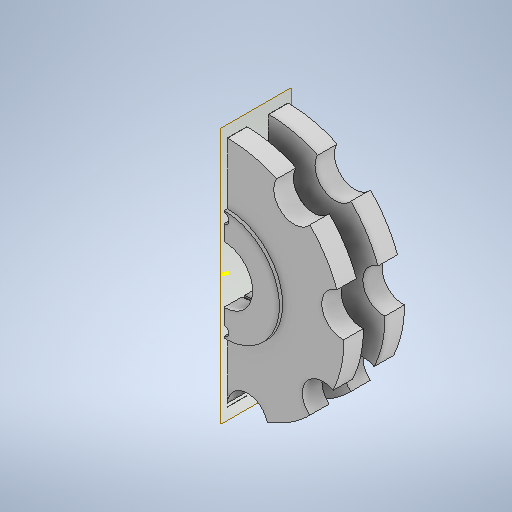
# Autodesk Inventor part: 59-01-002-C
Saved by Autodesk Inventor 2025.2 (Build 292293000, 293)
## iProperties
Created: 2024-11-14
Part Number: 59-01-002-C
Material: Generic
Document SubType Name: Modeling
Designer: Zvonko.Gabric
Density: 1 g/cm^3
Appearance: Default
Description: Stator
Author: Zvonko.Gabric
Autodesk Inventor part; units mm, degrees
ref_plane "XZ Plane" through (0, 0, 0) normal (0, 1, 0) x (-1, 0, 0)
ref_plane "XY Plane" through (0, 0, 0) normal (0, 0, 1) x (1, 0, 0)
sketch "Sketch1" plane through (0, 0, 0) normal (0, 1, 0) x (-1, 0, 0)
  line L0 (0, 0) -> (0, -37.3)
  line L1 (0, -37.3) -> (-71.75, -37.3)
  line L2 (-71.75, -37.3) -> (-71.75, -25.3)
  line L3 (-71.75, -25.3) -> (-41.05, -25.3)
  line L4 (-41.05, -25.3) -> (-41.05, -12)
  line L5 (-41.05, -12) -> (-71.75, -12)
  line L6 (-71.75, -12) -> (-71.75, 0)
  line L7 (-71.75, 0) -> (0, 0)
  dimension "d0" = 37.3
  dimension "d1" = 71.75
  dimension "d2" = 12
  dimension "d3" = 30.7
  dimension "d4" = 13.3
  constraints: 16 end point, 5 perpendicular, 2 point on line, 1 parallel, 1 vertical
  measures "d0" distance of L0.start L0.end
  measures "d1" distance of L0.end L1.end
  measures "d2" distance of L1.end L2.end
  measures "d3" distance of L2.end L3.end
  measures "d4" distance of L3.end L4.end
revolve "Revolution1" add sketch "Sketch1" angle 360 about axis through (0, 0, 0) along (0, 0, -1)
sketch "Sketch2" plane through (0, 0, 0) normal (0, 0, 1) x (1, 0, 0)
  circle A0 centre (0, 0) radius 34
  dimension "d6" = 68
  constraints: 1 centre point, 1 coincident
  measures "d6" diameter of A0
extrude "Extrusion1" add sketch "Sketch2" along normal blind 2
sketch "Sketch3" plane through (0, 0, 2) normal (0, 0, 1) x (1, 0, 0)
  circle A0 centre (0, 0) radius 17.5
  dimension "d9" = 35
  constraints: 1 centre point, 1 coincident
  measures "d9" diameter of A0
extrude "Extrusion2" cut sketch "Sketch3" against normal through all
sketch "Sketch4" plane through (0, 0, 2) normal (0, 0, 1) x (1, 0, 0)
  point P0 (0, 0)
sketch "Sketch7" plane through (0, 0, 0) normal (0, 0, 1) x (1, 0, 0)
  circle A0 centre (0, 0) radius 71.75
  circle A1 centre (-12.4593, 70.66) radius 12.5
  line L0 (-12.4593, 70.66) -> (0, 0) construction
  line L1 (0, 71.75) -> (0, 0) construction
  line L2 (-50.7349, 50.7349) -> (0, 0) construction
  circle A2 centre (-58.7742, 41.1541) radius 12.5
  line L3 (-71.75, 0) -> (0, 0) construction
  circle A3 centre (-70.66, -12.4593) radius 12.5
  line L4 (-50.7349, -50.7349) -> (0, 0) construction
  circle A4 centre (-41.1541, -58.7742) radius 12.5
  line L5 (0, -71.75) -> (0, 0) construction
  circle A5 centre (12.4593, -70.66) radius 12.5
  line L6 (50.7349, -50.7349) -> (0, 0) construction
  circle A6 centre (58.7742, -41.1541) radius 12.5
  line L7 (71.75, 0) -> (0, 0) construction
  circle A7 centre (70.66, 12.4593) radius 12.5
  line L8 (50.7349, 50.7349) -> (0, 0) construction
  circle A8 centre (41.1541, 58.7742) radius 12.5
  line L9 (41.1541, 58.7742) -> (0, 0) construction
  line L10 (70.66, 12.4593) -> (0, 0) construction
  dimension "d26" = 25
  dimension "d27" = 143.5
  dimension "d28" = 10
  dimension "d31" = 360
  constraints: 22 end point, 9 centre point, 3 coincident, 2 point on circle, 1 vertical, 39 other
  measures "d26" diameter of A1
  measures "d27" diameter of A0
  measures "d28" angle of L1 L0
extrude "Extrusion4" cut sketch "Sketch7" against normal through all contours A7 A0 | A0 A7 | A6 A0 | A0 A6 | A8 A0 | A0 A8 | A5 A0 | A0 A5 | A1 A0 | A0 A1 | A4 A0 | A0 A4 | A2 A0 | A0 A2 | A3 A0 | A0 A3
sketch "Sketch8" plane through (0, 0, 2) normal (0, 0, 1) x (1, 0, 0)
  arc A0 (30.3291, 65.0247) -> (-0.0069, 71.75) centre (0, 0) ccw projected
  line L0 (-0.0069, 71.75) -> (-0.0069, -34) construction
  circle A1 centre (0, 0) radius 34 projected
  circle A2 centre (-0.0069, 30) radius 3
  circle A3 centre (-0.0069, -30) radius 3
  dimension "d35" = 30
  dimension "d36" = 6
  dimension "d37" = 30
  dimension "d38" = 6
  constraints: 2 centre point, 2 end point, 2 point on line, 1 vertical, 2 other
  measures "d35" distance of point (0, 0) A3.centre
  measures "d36" diameter of A3
  measures "d37" distance of point (0, 0) A2.centre
  measures "d38" diameter of A2
extrude "Extrusion5" cut sketch "Sketch8" against normal blind 17 contours A2 | A3
thread "Thread1" size "M6x1" class "6H" standard "ANSI Metric M Profile" length 12
thread "Thread2" size "M6x1" class "6H" standard "ISO Metric profile" length 12 offset 5
thread "Thread3" size "M6x1" class "6H" standard "ISO Metric profile" length 12 offset 5
sketch "Sketch10" plane through (41.1541, 58.7742, 0) normal (0, 0, 1) x (0.819152, -0.5735764, 0)
  circle A0 centre (0, -71.75) radius 41.05 projected
  circle A1 centre (-17.2129, -47.1794) radius 3 projected
  line L0 (0, -71.75) -> (-17.2129, -47.1794) construction
  arc A2 (-41.1597, -130.5202) -> (-58.7702, -112.9097) centre (-50.7349, -122.4849) ccw projected
  line L1 (0, -71.75) -> (-50.7349, -122.4849) construction
  arc A3 (-37.3679, -113.3606) -> (-41.6106, -109.1179) centre (-39.4892, -111.2392) ccw
  arc A4 (-40.0331, -116.0257) -> (-44.2757, -111.7831) centre (-50.7349, -122.4849) ccw
  line L2 (-39.4892, -111.2392) -> (-37.3679, -113.3606) construction
  line L3 (-39.4892, -111.2392) -> (-41.6106, -109.1179) construction
  line L4 (-37.3679, -113.3606) -> (-40.0331, -116.0257)
  line L5 (-41.6106, -109.1179) -> (-44.2757, -111.7831)
  point P0 (-42.9431, -110.4505)
  point P1 (-44.2757, -111.7831)
  point P2 (-40.0331, -116.0257)
  dimension "d56" = 6
  dimension "d57" = 55
  dimension "d58" = 6
  constraints: 12 end point, 4 point on circle, 2 centre point, 1 coincident, 1 midpoint, 1 point on line, 1 tangent
  measures "d56" diameter of A3
  measures "d57" distance from line of L0 L2.start
  measures "d58" distance from line of point (-42.943, -110.451) L4
extrude "Extrusion7" cut sketch "Sketch10" against normal blind 13 contours A2 L5 A3 L4
sketch "Sketch11" plane through (-41.1541, -58.7742, 0) normal (0, 0, 1) x (0.819152, -0.5735764, 0)
  circle A0 centre (-17.2129, 96.3206) radius 3 projected
  line L0 (0, 71.75) -> (-17.2129, 96.3206) construction
  line L1 (0, 71.75) -> (-36.8559, 45.9306) construction
  circle A1 centre (-36.8559, 45.9306) radius 2.05
  dimension "d61" = 4.1
  dimension "d62" = 45
  constraints: 4 end point, 1 centre point, 1 coincident
  measures "d61" diameter of A1
  measures "d62" distance from line of L0 A1.centre
extrude "Extrusion8" cut sketch "Sketch11" against normal blind 8 contours A1
sketch "Sketch12" plane through (41.1541, 58.7742, -37.3) normal (0, 0, -1) x (-0.819152, 0.5735764, 0)
  circle A0 centre (0, -71.75) radius 31
  dimension "d65" = 62
  constraints: 1 centre point, 1 coincident
  measures "d65" diameter of A0
extrude "Extrusion9" cut sketch "Sketch12" against normal blind 5.5
chamfer "Chamfer1" distance 10 distance2 5.5 1 edges at (25.3937, -17.7809, -37.3) measured on face at (49.9559, -10.1171, -37.3)
sketch "Sketch13" plane through (-0.0069, 30, -15) normal (0, 0, 1) x (1, 0, 0)
  point P0 (0.0069, -30)
sketch "Sketch14" plane through (-0.0069, 30, -15) normal (0, 0, 1) x (1, 0, 0)
  point P0 (0.0069, -30)
ref_plane "Work Plane1" through (0, 0, 0) normal (1, 0, 0) x (0, 1, 0)
sketch "Sketch15" plane through (0, 0, 0) normal (1, 0, 0) x (0, 1, 0)
  point P0 (0, 0)
sketch "Sketch16" plane through (0, 0, 0) normal (1, 0, 0) x (0, 1, 0)
  line L0 (27, -15) -> (33, -15) projected
  line L1 (30, -15) -> (30, -17)
  line L2 (30, -17) -> (33, -15)
  line L3 (-33, -15) -> (-27, -15) projected
  line L4 (-30, -15) -> (-30, -17)
  line L5 (-30, -17) -> (-27, -15)
  point P0 (0, 0)
  dimension "d72" = 2
  dimension "d73" = 2
  constraints: 8 end point, 2 midpoint, 2 vertical
  measures "d72" distance of L1.start L1.end
  measures "d73" distance of L4.start L4.end
revolve "Revolution2" cut sketch "Sketch16" angle 360 about axis through (0, 30, -15) along (0, 0, -1) contours L0 L2 L1
sketch "Sketch17" plane through (0, 0, 0) normal (1, 0, 0) x (0, 1, 0)
  line L0 (-33, -15) -> (-27, -15) projected
  line L1 (-30, -15) -> (-30, -17)
  line L2 (-30, -17) -> (-27, -15)
  point P0 (0, 0)
  dimension "d75" = 2
  constraints: 4 end point, 1 midpoint, 1 vertical
  measures "d75" distance of L1.start L1.end
revolve "Revolution3" cut sketch "Sketch17" angle 360 about axis through (0, -30, -15) along (0, 0, -1)
sketch "Sketch18" plane through (0, 0, 0) normal (1, 0, 0) x (0, 1, 0)
  point P0 (0, 0)
sketch "Sketch19" plane through (0, 0, 0) normal (1, 0, 0) x (0, 1, 0)
  line L0 (-17.5, 2) -> (-17.5, -31.8) projected
  line L1 (-17.5, -20.8) -> (-18.5, -20.8)
  line L2 (-18.5, -20.8) -> (-18.5, -19.2)
  line L3 (-18.5, -19.2) -> (-17.5, -19.2)
  line L4 (0, -14.9) -> (0, -39.226) construction
  line L5 (31, -31.8) -> (-31, -31.8) projected
  point P0 (0, 0)
  point P1 (-18, -20.8)
  dimension "d77" = 1.6
  dimension "d78" = 11
  dimension "d79" = 1
  constraints: 8 end point, 2 perpendicular, 2 point on line, 1 horizontal, 1 midpoint, 1 vertical
  measures "d77" distance of L1.end L2.end
  measures "d78" distance from line of point (-18, -20.8) L5
  measures "d79" distance between parallel lines of L0 L2
revolve "Revolution4" cut sketch "Sketch19" angle 360 about axis through (0, 0, -14.9) along (0, 0, -1)
sketch "Sketch20" plane through (0, 0, 0) normal (1, 0, 0) x (0, 1, 0)
  line L0 (-17.1194, -9) -> (-18.5, -9)
  line L1 (-18.5, -9) -> (-18.5, -10.6)
  line L2 (-18.5, -10.6) -> (-17.1194, -10.6)
  line L3 (-17.1194, -10.6) -> (-17.1194, -9)
  line L4 (34, 2) -> (-34, 2) projected
  line L5 (0.0069, -14.9986) -> (0.0069, -6.8686)
  line L6 (0.0069, -12) -> (0.0069, 0) projected
  line L7 (-18.5, -20.8) -> (-18.5, -19.2) projected
  line L8 (-18.5, -20) -> (-18.5, -11.367) construction
  point P0 (0, 0)
  dimension "d86" = 1.6
  dimension "d87" = 0
  dimension "d89" = 11
  constraints: 12 end point, 2 parallel, 1 horizontal, 1 midpoint, 1 perpendicular, 1 point on line, 1 vertical
  measures "d86" distance of L2.end L0.start
  measures "d87" distance between parallel lines of L1 L8
  measures "d89" distance between parallel lines of L4 L0
revolve "Revolution6" cut sketch "Sketch20" angle 360 about axis through (0, 0.0069, -14.9986) along (0, 0, 1)
body "Solid1"
